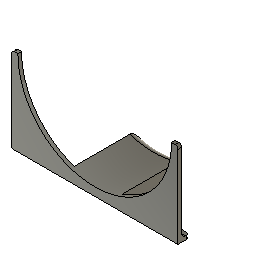
design (Autodesk Fusion 360 design; units mm, degrees)
Autodesk Fusion 360 part; units mm, degrees
sketch "Sketch1" plane through (0, 0, 0) normal (0, 1, 0) x (1, 0, 0) in component "Component"
  circle A0 centre (0, 0) radius 20.75
  line L0 (-22.5, 23) -> (22.5, 23)
  line L1 (0, 0) -> (0, 23) construction
  line L2 (-22.5, 23) -> (-22.5, 0)
  line L3 (22.5, 23) -> (22.5, 0)
  line L4 (-22.5, 0) -> (22.5, 0)
  line L5 (6.5, 19.7056) -> (6.5, 23)
  line L6 (-6.5, 19.7056) -> (-6.5, 23)
  line L7 (-22.5, 22) -> (22.5, 22)
  dimension "d1" = 41.5
  dimension "d2" = 45
  dimension "d3" = 23
  dimension "d4" = 13
  dimension "d9" = 1
  constraint coincident A0.centre L1.start
  constraint horizontal L0
  constraint coincident L0 L1.end
  constraint perpendicular L0 L1
  constraint midpoint L0 L1.end
  constraint perpendicular L0 L2
  constraint perpendicular L0 L3
  constraint perpendicular L3 L4
  constraint coincident A0.centre L4
  constraint coincident A0 L5.start
  constraint coincident L0 L5.end
  constraint perpendicular L0 L5
  constraint coincident A0 L6.start
  constraint coincident L0 L6.end
  constraint perpendicular L0 L6
  constraint symmetric L1 L5 L6
  constraint coincident L2 L7.start
  constraint coincident L3 L7.end
  constraint perpendicular L3 L7
  measures "d1" diameter of A0
  measures "d2" distance of L0.start L0.end
  measures "d3" distance of A0.centre L0
  measures "d4" distance of L5 L6
  measures "d9" distance of L0 L7
extrude "Extrude1" add sketch "Sketch1" along normal blind 1 contours A0 L3 L4 L5 L7 | A0 L2 L4 L6 L7 | L0 L3 L5 L7 | L0 L2 L6 L7 makes body 1 at (13.5543, 0, -21.0541) makes body 2 at (-13.5543, 0, -21.0541) in component "Component"
extrude "Extrude2" add sketch "Sketch1" along normal blind 18 contours A0 L5 L6 L7 | L0 L5 L6 L7 bodies 1 2 in component "Component"
extrude "Extrude3" add sketch "Sketch1" along normal blind 3 contours L0 L3 L5 L7 | L0 L2 L6 L7 bodies 1 in component "Component"
fillet "Fillet1" radius 2 3 edges at (0, 18, -20.75) (6.5, 18, -21.3528) (-6.5, 18, -21.3528) on bodies 1 in component "Component"
fillet "Fillet2" radius 0.75 4 edges at (22.5, 0.5, 0) (-22.5, 0.5, 0) (22.5, 3, -22.5) (-22.5, 3, -22.5) on bodies 1 in component "Component"
fillet "Fillet3" radius 1 2 edges at (14.5, 1, -22) (-14.5, 1, -22) on bodies 1 in component "Component"
component "Component" placed x (1, 0, 0) y (0, 1, 0) z (0, 0, 1) at (0, 0, 0)
